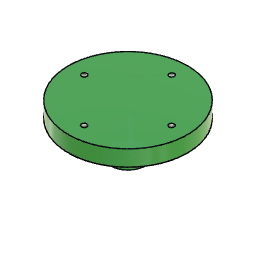
Braço robótico 3.0(Suporte para o braço, parte 1) v7 (Autodesk Fusion 360 design; units mm, degrees)
Autodesk Fusion 360 part; units mm, degrees
note: some values were not read from the file. Set by a fixed rule: which sketch regions a step uses.
sketch "Sketch1" plane through (0, 0, 0) normal (0, 0, 1) x (1, 0, 0)
  circle A0 centre (0, 0) radius 37.5
  dimension "d1" = 75
  constraint coincident A0.centre origin
  measures "d1" diameter of A0
extrude "Extrude1" add sketch "Sketch1" along normal blind 10
sketch "Sketch2" plane through (0, 0, 0) normal (0, 0, -1) x (1, 0, 0)
  circle A0 centre (0, 0) radius 37.5
  circle A1 centre (0, 0) radius 10.985
  dimension "d4" = 21.97
  constraint concentric A0 A1
  measures "d4" diameter of A1
extrude "Extrude2" add sketch "Sketch2" along normal blind 20.3 contours A1
sketch "Sketch3" plane through (0, 0, -20.3) normal (0, 0, -1) x (1, 0, 0)
  circle A0 centre (0, 0) radius 10.985
  circle A1 centre (0, 0) radius 2.5
  dimension "d7" = 5
  constraint coincident A0.centre A1.centre
  measures "d7" diameter of A1
extrude "Extrude3" cut sketch "Sketch3" against normal blind 20.3 contours A1
sketch "Sketch5" plane through (0, 0, -20.3) normal (0, 0, -1) x (1, 0, 0)
  circle A0 centre (0, 0) radius 2.5
  circle A1 centre (0, 0) radius 10.985
  line L0 (0, -1.992) -> (1.5106, -1.992)
  line L1 (0, -1.992) -> (-1.5106, -1.992)
  circle A2 centre (0, 0) radius 2.5
  constraint coincident A0 L0.end
  constraint coincident A0 L1.end
  constraint concentric A0 A2
extrude "Extrude4" add sketch "Sketch5" against normal blind 20.3 contours A0 L0 L1 A2 picked at (0, -2.3263)
sketch "Sketch6" plane through (0, 1.992, 0) normal (0, -1, 0) x (1, 0, 0)
  line L0 (-1.5106, -20.3) -> (1.5106, -20.3)
  line L1 (1.5106, -20.3) -> (1.5106, 0)
  line L2 (1.5106, 0) -> (-1.5106, 0)
  line L3 (-1.5106, 0) -> (-1.5106, -20.3)
sketch "Sketch7" plane through (0, 0, -20.3) normal (0, 0, -1) x (1, 0, 0)
  arc A0 (1.5106, -1.992) -> (-1.5106, -1.992) centre (0, 0) ccw
  line L0 (1.5106, -1.992) -> (-1.5106, -1.992)
  circle A1 centre (0, 0) radius 10.985
hole "Hole1" at (0, 10.985, -13.2045) direction (0, -1, 0) diameter 2.175 depth 50 tip angle 180 counterbore diameter 5 counterbore depth 3
thread "Thread1" "ISO Metric profile 2.6 M2.6x0.45 6H"
sketch "Sketch8" plane through (0, 0, 10) normal (0, 0, 1) x (-1, 0, 0)
  circle A0 centre (0, 0) radius 37.5
sketch "Sketch9" plane through (0, 0, 10) normal (0, 0, 1) x (-1, 0, 0)
  circle A0 centre (0, 0) radius 37.5
  line L0 (-0.0392, -37.5) -> (-0.0278, -27.5)
  line L1 (37.5, -0.0392) -> (27.5, -0.0278)
  line L2 (0.0392, 37.5) -> (0.0278, 27.5)
  line L3 (-37.5, 0.0392) -> (-27.5, 0.0278)
  dimension "d19" = 10
  dimension "d21" = 360
  constraint coincident A0 L0.start
  measures "d19" distance of L0.start L0.end
hole "Hole2" at (0.0278, 27.5, 10) at (27.5, -0.0278, 10) at (-0.0278, -27.5, 10) at (-27.5, 0.0278, 10) direction (0, 0, -1) diameter 3.332 depth 50 tip angle 180
thread "Thread2" "ISO Metric profile 4.0 M4x0.7 6H"
component "6627T91_Stepper Motor" placed x (1, 0, 0) y (0, 1, 0) z (0, 0, 1) at (52.5447, 49.4652, -3.0795)
